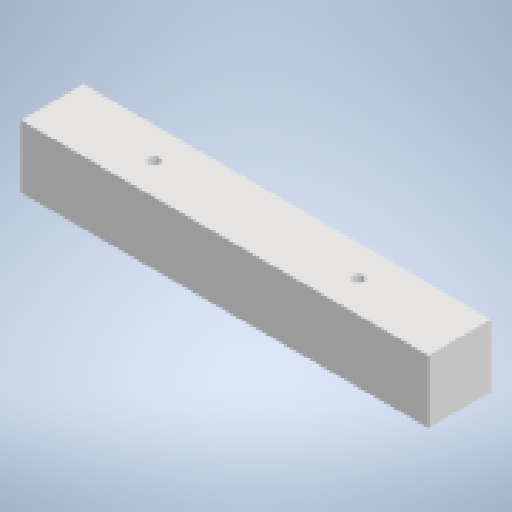
# Autodesk Inventor part: 3D지지대
Saved by Autodesk Inventor 2024 (Build 280153000, 153)
## iProperties
Created: 2024-04-09
Part Number: 3D지지대
Material: 일반
Document SubType Name: Modeling
Designer: ckhye
Density: 1 g/cm^3
Appearance: 기본값
Author: ckhye
Autodesk Inventor part; units mm, degrees
ref_plane "YZ Plane" through (0, 0, 0) normal (1, 0, 0) x (0, 1, 0)
ref_plane "XZ Plane" through (0, 0, 0) normal (0, 1, 0) x (-1, 0, 0)
ref_plane "XY Plane" through (0, 0, 0) normal (0, 0, 1) x (1, 0, 0)
sketch "스케치2" plane through (0, 0, 0) normal (0, 1, 0) x (-1, 0, 0)
  line L0 (65, 10) -> (-65, 10)
  line L1 (-65, 10) -> (-65, -10)
  line L2 (-65, -10) -> (65, -10)
  line L3 (65, -10) -> (65, 10)
  line L4 (65, 10) -> (-65, -10) construction
  line L5 (-65, 10) -> (65, -10) construction
  point P0 (0, 0)
  dimension "d2" = 130
  dimension "d4" = 20
  constraints: 12 end point, 2 midpoint, 2 parallel, 1 horizontal, 1 perpendicular
  measures "d2" distance of L2.end L1.end
  measures "d4" distance between parallel lines of L2 L0
extrude "돌출2" add sketch "스케치2" along normal blind 20
sketch "스케치3" plane through (0, 20, 0) normal (0, 1, 0) x (1, 0, 0)
  point P0 (0, 0)
  point P1 (32.5, 0)
  point P2 (-32.5, 0)
  dimension "d7" = 32.5
  dimension "d8" = 32.5
  measures "d7" distance of point (0, 0) point (32.5, 0)
  measures "d8" distance of point (0, 0) point (-32.5, 0)
hole "구멍1" at (32.5, 20, 0) at (-32.5, 20, 0) direction (0, -1, 0) diameter 3.5 end through all
equation "\"d8\" = d7"
